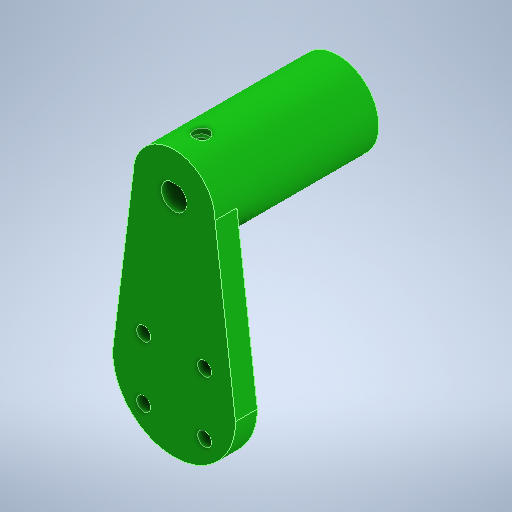
# Autodesk Inventor part: pen_holder
Saved by Autodesk Inventor 2025 (Build 290162000, 162)
## iProperties
Created: 2024-08-22
Part Number: pen_holder
Material: LCP Plastic
Document SubType Name: Modeling
Designer: pedro
Density: 1.626 g/cm^3
Appearance: Dark Green
Author: pedro
Autodesk Inventor part; units mm, degrees
ref_plane "YZ Plane" through (0, 0, 0) normal (1, 0, 0) x (0, 1, 0)
ref_plane "XZ Plane" through (0, 0, 0) normal (0, 1, 0) x (-1, 0, 0)
ref_plane "XY Plane" through (0, 0, 0) normal (0, 0, 1) x (1, 0, 0)
sketch "Sketch1" plane through (0, 0, 0) normal (0, 0, 1) x (1, 0, 0)
  arc A0 (-22.5, 0) -> (22.5, 0) centre (0, 0) ccw
  circle A1 centre (-11.14, 11.14) radius 2.5
  circle A2 centre (-11.14, -11.14) radius 2.5
  circle A3 centre (11.14, -11.14) radius 2.5
  circle A4 centre (11.14, 11.14) radius 2.5
  arc A5 (15, 60) -> (-15, 60) centre (0, 60) ccw
  line L0 (22.5, 0) -> (15, 60)
  line L1 (-22.5, 0) -> (-15, 60)
  dimension "d0" = 45
  dimension "d3" = 5
  dimension "d4" = 11.14
  dimension "d5" = 11.14
  dimension "d8" = 360
  dimension "d29" = 30
  constraints: 6 centre point, 4 end point, 4 point on circle, 1 coincident, 9 other
  measures "d0" diameter of A0
  measures "d3" diameter of A1
  measures "d4" horizontal distance of A0.centre A1.centre
  measures "d5" horizontal distance of A0.centre A1.centre
  measures "d29" diameter of A5
extrude "Extrusion1" add sketch "Sketch1" along normal blind 8
sketch "Sketch5" plane through (0, 0, 8) normal (0, 0, 1) x (1, 0, 0)
  arc A0 (15, 60) -> (-15, 60) centre (0, 60) ccw projected
  circle A1 centre (0, 60) radius 15
  point P0 (0, 0)
  point P1 (-15, 60)
  constraints: 1 centre point, 1 coincident
extrude "Extrusion3" add sketch "Sketch5" against normal blind 60
sketch "Sketch6" plane through (0, 0, 8) normal (0, 0, 1) x (1, 0, 0)
  arc A0 (15, 60) -> (-15, 60) centre (0, 60) ccw projected
  arc A1 (-1.8762, 64.2) -> (1.8762, 64.2) centre (0, 60) ccw
  line L0 (-1.8762, 64.2) -> (1.8762, 64.2)
  point P0 (0, 0)
  point P1 (0, 55.4)
  point P2 (0, 64.2)
  dimension "d32" = 9.2
  dimension "d39" = 8.8
  constraints: 3 point on circle, 2 end point, 1 centre point, 1 coincident, 1 horizontal, 1 midpoint
  measures "d32" diameter of A1
  measures "d39" distance of point (0, 55.4) point (0, 64.2)
extrude "Extrusion4" cut sketch "Sketch6" against normal through all
ref_plane "Work Plane2" through (0, 75, 8) normal (0, 1, 0) x (-1, 0, 0)
sketch "Sketch7" plane through (0, 75, 8) normal (0, 1, 0) x (-1, 0, 0)
  circle A0 centre (0, -10) radius 1.35
  line L0 (15, 0) -> (-15, 0) projected
  point P0 (0, -8)
  point P1 (0, 0)
  dimension "d35" = 2.7
  dimension "d36" = 10
  constraints: 1 centre point, 1 midpoint
  measures "d35" diameter of A0
  measures "d36" distance of point (0, 0) A0.centre
extrude "Extrusion5" cut sketch "Sketch7" against normal blind 15
sketch "Sketch8" plane through (0, 75, 8) normal (0, 1, 0) x (-1, 0, 0)
  circle A0 centre (0, -10) radius 1.35 projected
  circle A1 centre (0, -10) radius 2.75
  point P0 (0, -8)
  dimension "d40" = 5.5
  constraints: 1 centre point, 1 coincident
  measures "d40" diameter of A1
extrude "Extrusion6" cut sketch "Sketch8" against normal blind 2
body "Solid1"
